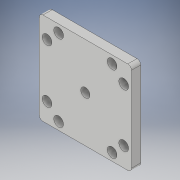
# Autodesk Inventor part: 20_IM_LED_holder
Saved by Autodesk Inventor 2019 (Build 230136000, 136)
## iProperties
Created: 2020-10-28
Part Number: 20_IM_LED_holder
Material: Generic
Document SubType Name: Modeling
Designer: wanghaoran
Density: 1 g/cm^3
Appearance: Default
Author: wanghaoran
Autodesk Inventor part; units mm, degrees
ref_plane "YZ Plane" through (0, 0, 0) normal (1, 0, 0) x (0, 1, 0)
ref_plane "XZ Plane" through (0, 0, 0) normal (0, 1, 0) x (-1, 0, 0)
ref_plane "XY Plane" through (0, 0, 0) normal (0, 0, 1) x (1, 0, 0)
sketch "Sketch1" plane through (0, 0, 0) normal (0, 0, 1) x (1, 0, 0)
  line L0 (-25, 25) -> (25, 25)
  line L1 (25, 25) -> (25, -25)
  line L2 (25, -25) -> (-25, -25)
  line L3 (-25, -25) -> (-25, 25)
  line L4 (-25, 25) -> (25, -25) construction
  line L5 (25, 25) -> (-25, -25) construction
  circle A0 centre (0, 0) radius 2.5
  circle A1 centre (-20.8, -14.5) radius 2.65
  circle A2 centre (-14.5, -20.8) radius 2.65
  circle A3 centre (-20.8, 14.5) radius 2.65
  circle A4 centre (20.8, -14.5) radius 2.65
  circle A5 centre (20.8, 14.5) radius 2.65
  circle A6 centre (-14.5, 20.8) radius 2.65
  circle A7 centre (14.5, -20.8) radius 2.65
  circle A8 centre (14.5, 20.8) radius 2.65
  dimension "d0" = 50
  dimension "d1" = 50
  dimension "d2" = 5
  dimension "d5" = 5.3
  dimension "d6" = 4.2
  dimension "d8" = 10.5
  dimension "d11" = 29
  dimension "d14" = 41.6
  constraints: 12 end point, 9 centre point, 4 symmetric about line, 2 horizontal, 2 midpoint, 2 parallel, 1 coincident, 1 perpendicular, 1 vertical, 10 other
  measures "d0" distance of L1.end L2.end
  measures "d1" distance of L0.end L1.end
  measures "d2" diameter of A0
  measures "d5" diameter of A1
  measures "d6" distance from line of A1.centre L3
  measures "d8" distance from line of L2 A1.centre
  measures "d11" distance of A1.centre A3.centre
  measures "d14" distance of A1.centre A4.centre
extrude "Extrusion1" add sketch "Sketch1" along normal blind 5
fillet "Fillet1" radius 2 4 edges at (-25, 25, 2.5) (25, 25, 2.5) (-25, -25, 2.5) (25, -25, 2.5)
body "Solid1"
